Autodesk Fusion 360 part; units mm, degrees
note: some values were not read from the file. Chosen so that the rebuilt part matches the saved one: which bodies a step acts on. Set by a fixed rule: which sketch regions a step uses.
(part 3 of 3)
sketch "Sketch8" plane through (0, 0.6486, 0) normal (0, 1, 0) x (1, 0, 0)
  line L0 (0.635, 0) -> (-0.635, 0)
  line L1 (-0.635, 0) -> (-0.635, 1.947)
  line L2 (-0.635, 1.947) -> (0.635, 1.947)
  line L3 (0.635, 1.947) -> (0.635, 0)
  line L4 (0.1879, 0.6932) -> (0.1773, 0.6456)
  line L5 (-0.3149, 1.0213) -> (-0.3096, 1.0054)
  line L6 (-0.3307, 0.5821) -> (-0.3254, 0.6085)
  line L7 (-0.4948, 0.598) -> (-0.8334, 0.2593)
  line L8 (-0.1773, 0.5556) -> (-0.172, 0.598)
  line L9 (-0.3254, 0.6297) -> (-0.3307, 0.6509)
  line L10 (-0.4101, 0) -> (-0.2831, 0.1005)
  line L11 (-0.4683, 1.0425) -> (-0.4683, 1.0054)
  line L12 (-0.2831, 0.1005) -> (-0.2831, 0.2064)
  line L13 (-0.2778, 0.3069) -> (-0.1931, 0.508)
  line L14 (-0.172, 0.6456) -> (-0.1826, 0.6932)
  line L15 (-0.4207, 0.3598) -> (-0.2778, 0.3069)
  line L16 (-0.4683, 1.0054) -> (-0.4577, 0.9631)
  line L17 (-0.3149, 1.0425) -> (-0.3149, 1.0213)
  line L18 (-0.336, 0.5609) -> (-0.3307, 0.5821)
  line L19 (13.8033, 2.0479) -> (13.8033, 2.3548)
  line L20 (0.4207, 2.8522) -> (0.4207, 2.5347)
  line L21 (0.3836, 2.8152) -> (0.4207, 2.8522)
  line L22 (0.4948, 2.8628) -> (0.4789, 2.8734)
  line L23 (13.5229, 2.831) -> (13.5229, 2.8416)
  line L24 (0.9075, 2.9686) -> (1.0081, 2.7675)
  line L25 (13.6022, 2.7675) -> (13.6022, 2.4871)
  line L26 (0.8811, 2.8522) -> (0.9181, 2.8152)
  line L27 (13.5811, 2.7675) -> (13.6022, 2.7675)
  line L28 (0.5689, 2.9686) -> (0.3942, 2.9686)
  line L29 (0.5054, 2.8416) -> (0.4948, 2.8628)
  line L30 (0.8811, 2.8522) -> (0.8811, 2.5347)
  line L31 (13.6022, 2.323) -> (13.6022, 2.0479)
  line L32 (13.5281, 2.3548) -> (13.5281, 2.0479)
  line L33 (13.5281, 2.8205) -> (13.5281, 2.5135)
  line L34 (1.0081, 2.7675) -> (0.9763, 2.7675)
  line L35 (0.5847, 2.7675) -> (0.5636, 2.7675)
  line L36 (0.8387, 2.8787) -> (0.8229, 2.8734)
  line L37 (0.336, 2.7675) -> (0.3254, 2.7675)
  line L38 (13.4805, 2.8787) -> (13.4964, 2.8734)
  line L39 (13.8086, 2.8416) -> (13.8033, 2.831)
  line L40 (0.7382, 2.7675) -> (0.717, 2.7675)
  line L41 (0.4789, 2.8734) -> (0.463, 2.8787)
  line L42 (13.8086, 2.3654) -> (13.8086, 2.0479)
  line L43 (13.507, 2.8628) -> (13.5229, 2.8416)
  line L44 (13.4382, 2.8522) -> (13.4382, 2.5347)
  line L45 (0.5054, 2.8416) -> (0.5159, 2.8205)
  line L46 (0.3254, 2.7675) -> (0.3254, 2.4871)
  line L47 (0.5265, 2.7993) -> (0.5159, 2.8205)
  line L48 (13.3482, 2.7675) -> (13.3641, 2.7781)
  line L49 (0.9763, 2.0479) -> (0.9763, 2.323)
  line L50 (2.3892, 2.2013) -> (2.3892, 2.0479)
  line L51 (1.5161, 2.0479) -> (1.5161, 2.2013)
  line L52 (13.9674, 2.7781) -> (13.9832, 2.7675)
  line L53 (4.1196, 2.2013) -> (4.1196, 2.0479)
  line L54 (13.3376, 2.4871) -> (13.3376, 2.7675)
  line L55 (6.7231, 2.0479) -> (6.2944, 2.0479)
  line L56 (0.5054, 2.8416) -> (0.5054, 2.5241)
  line L57 (7.5962, 2.2013) -> (7.5962, 2.0479)
  line L58 (1.0874, 2.2013) -> (1.0874, 2.0479)
  line L59 (2.8178, 2.2013) -> (2.3892, 2.2013)
  line L60 (7.157, 1.4129) -> (7.157, 2.4395)
  line L61 (0.717, 2.7675) -> (0.5847, 2.7675)
  line L62 (1.5161, 2.2013) -> (1.0874, 2.2013)
  line L63 (8.0248, 2.2013) -> (7.5962, 2.2013)
  line L64 (13.3059, 2.4871) -> (13.3059, 2.7675)
  line L65 (10.6283, 2.2013) -> (10.1944, 2.2013)
  line L66 (0.4207, 2.3707) -> (0.4207, 2.0479)
  line L67 (0.8811, 2.3707) -> (0.8811, 2.0479)
  line L68 (2.8178, 2.0479) -> (2.8178, 2.2013)
  line L69 (0.5159, 2.0479) -> (0.5159, 2.3548)
  line L70 (0.3254, 2.323) -> (0.3254, 2.0479)
  line L71 (13.5229, 2.8416) -> (13.5229, 2.5241)
  line L72 (13.3059, 2.7675) -> (13.3376, 2.7675)
  line L73 (0.7858, 2.8205) -> (0.7858, 2.5135)
  line L74 (0.7964, 2.3654) -> (0.7964, 2.0479)
  line L75 (6.7231, 2.2013) -> (6.7231, 2.0479)
  line L76 (11.4961, 2.0479) -> (11.4961, 2.2013)
  line L77 (0.717, 1.8097) -> (0.5001, 1.5928)
  line L78 (0.7911, 1.5187) -> (0.6535, 2.0479)
  line L79 (0.717, 2.323) -> (0.717, 2.0479)
  line L80 (0.3836, 2.3495) -> (0.3836, 2.0479)
  line L81 (10.6283, 2.0479) -> (10.1944, 2.0479)
  line L82 (5.4213, 2.2013) -> (4.9927, 2.2013)
  line L83 (0.5159, 2.5135) -> (0.5159, 2.8205)
  line L84 (13.4117, 2.9686) -> (13.5864, 2.9686)
  line L85 (13.3376, 2.0479) -> (13.3376, 2.323)
  line L86 (8.0248, 2.0479) -> (7.5962, 2.0479)
  line L87 (13.4594, 2.8734) -> (13.4805, 2.8787)
  line L88 (4.1196, 2.0479) -> (3.6909, 2.0479)
  line L89 (3.6909, 2.2013) -> (3.6909, 2.0479)
  line L90 (0.5054, 2.3654) -> (0.5054, 2.0479)
  line L91 (13.3376, 2.7675) -> (13.3482, 2.7675)
  line L92 (0.9181, 2.0479) -> (0.9181, 2.3495)
  line L93 (0.7858, 2.3548) -> (0.7858, 2.0479)
  line L94 (13.7716, 2.7781) -> (13.8033, 2.8205)
  line L95 (1.0081, 2.0479) -> (1.0081, 2.323)
  line L96 (0.8229, 2.8734) -> (0.807, 2.8628)
  line L97 (13.2318, 2.2013) -> (12.7979, 2.2013)
  line L98 (12.7979, 2.2013) -> (12.7979, 2.0479)
  line L99 (13.5229, 2.3654) -> (13.5229, 2.0479)
  line L100 (13.4011, 2.0479) -> (13.4011, 2.3495)
  line L101 (13.8086, 2.8416) -> (13.8086, 2.5241)
  line L102 (8.8979, 2.2013) -> (9.3266, 2.2013)
  line L103 (13.5281, 2.8205) -> (13.5229, 2.831)
  line L104 (0.7858, 2.8205) -> (0.7964, 2.8416)
  line L105 (0.3678, 2.794) -> (0.3519, 2.7781)
  line L106 (4.1196, 2.2013) -> (3.6909, 2.2013)
  line L107 (0.8811, 2.8522) -> (0.8599, 2.8734)
  line L108 (13.3059, 2.0479) -> (13.3059, 2.323)
  line L109 (9.3266, 2.0479) -> (8.8979, 2.0479)
  line L110 (6.2944, 2.2013) -> (6.2944, 2.0479)
  line L111 (13.7504, 2.7675) -> (13.7716, 2.7781)
  line L112 (13.2318, 2.0479) -> (12.7979, 2.0479)
  line L113 (0.3836, 2.8152) -> (0.3678, 2.794)
  line L114 (13.6022, 2.7675) -> (13.7292, 2.7675)
  line L115 (0.9763, 2.4871) -> (0.9763, 2.7675)
  line L116 (0.717, 2.7675) -> (0.717, 2.4871)
  line L117 (0.3836, 2.8152) -> (0.3836, 2.5135)
  line L118 (0.7594, 2.7781) -> (0.7382, 2.7675)
  line L119 (13.4382, 2.3707) -> (13.4382, 2.0479)
  line L120 (0.9181, 2.5135) -> (0.9181, 2.8152)
  line L121 (13.8033, 2.5135) -> (13.8033, 2.8205)
  line L122 (13.4011, 2.5135) -> (13.4011, 2.8152)
  line L123 (13.8033, 2.831) -> (13.8033, 2.8205)
  line L124 (0.9657, 2.7675) -> (0.9181, 2.8152)
  line L125 (0.463, 2.8787) -> (0.4419, 2.8681)
  line L126 (13.4382, 2.8522) -> (13.4594, 2.8734)
  line L127 (11.9301, 2.0479) -> (11.4961, 2.0479)
  line L128 (13.2318, 2.2013) -> (13.2318, 2.0479)
  line L129 (0.807, 2.8628) -> (0.7964, 2.8416)
  line L130 (1.0081, 2.4871) -> (1.0081, 2.7675)
  line L131 (0.9075, 2.9686) -> (0.7329, 2.9686)
  line L132 (13.544, 2.7993) -> (13.5599, 2.7781)
  line L133 (13.7292, 2.7675) -> (13.7504, 2.7675)
  line L134 (0.5477, 2.7781) -> (0.5265, 2.7993)
  line L135 (0.3519, 2.7781) -> (0.336, 2.7675)
  line L136 (13.417, 2.8363) -> (13.4011, 2.8152)
  line L137 (0.7752, 2.7993) -> (0.7594, 2.7781)
  line L138 (13.8086, 2.8416) -> (13.8245, 2.8628)
  line L139 (0.4419, 2.8681) -> (0.4207, 2.8522)
  line L140 (0.9763, 2.7675) -> (0.9657, 2.7675)
  line L141 (13.4964, 2.8734) -> (13.507, 2.8628)
  line L142 (13.4382, 2.8522) -> (13.417, 2.8363)
  line L143 (13.5599, 2.7781) -> (13.5811, 2.7675)
  line L144 (0.7964, 2.8416) -> (0.7964, 2.5241)
  line L145 (0.5636, 2.7675) -> (0.5477, 2.7781)
  line L146 (0.7858, 2.8205) -> (0.7752, 2.7993)
  line L147 (13.5281, 2.8205) -> (13.544, 2.7993)
  line L148 (0.8599, 2.8734) -> (0.8387, 2.8787)
  line L149 (0.3201, 1.0425) -> (0.3201, 1.8415)
  line L150 (-0.4948, 1.6827) -> (-0.8334, 1.3494)
  line L151 (0.2831, 0.1005) -> (0.2831, 0.2064)
  line L152 (-0.336, 0.5609) -> (-0.4207, 0.3598)
  line L153 (0.2778, 0.3069) -> (0.1931, 0.508)
  line L154 (0.5001, 0.2064) -> (0.5001, 1.9473)
  line L155 (-0.8334, 0) -> (-0.8334, 2.0479)
  line L156 (15.1527, 2.0479) -> (15.1527, 0)
  line L157 (-0.463, 0.9684) -> (-0.3307, 0.6509)
  line L158 (-0.4948, 1.3229) -> (-0.8334, 0.9843)
  line L159 (-0.1879, 0.508) -> (-0.1773, 0.5556)
  line L160 (-0.3254, 0.6085) -> (-0.3254, 0.6297)
  line L161 (-0.4948, 0.9631) -> (-0.8334, 0.6244)
  line L162 (-0.1826, 0.6932) -> (-0.3096, 1.0054)
  line L163 (-0.172, 0.598) -> (-0.172, 0.6456)
  line L164 (0.1773, 0.598) -> (0.1826, 0.5556)
  line L165 (0.1773, 0.6456) -> (0.1773, 0.598)
  line L166 (0.2831, 0.1005) -> (-0.2831, 0.1005)
  line L167 (-0.3149, 1.2806) -> (-0.4683, 1.2806)
  line L168 (-0.4948, 0.2381) -> (-0.7329, 0)
  line L169 (0.1826, 0.5556) -> (0.1931, 0.508)
  line L170 (0.336, 0.6509) -> (0.3307, 0.6297)
  line L171 (7.157, -0.381) -> (7.157, 0.6456)
  line L172 (-0.4948, 0.2064) -> (-0.4948, 1.9473)
  line L173 (0.7911, 1.524) -> (0.5001, 1.2277)
  line L174 (0.6482, 0.5345) -> (0.7911, 1.5187)
  line L175 (0.4736, 1.8415) -> (0.4736, 1.0425)
  line L176 (0.3201, 1.0213) -> (0.3201, 1.0425)
  line L177 (13.8245, 2.8628) -> (13.8351, 2.8734)
  line L178 (0.6694, 0.6773) -> (0.5001, 0.508)
  line L179 (-0.3149, 1.0425) -> (-0.3149, 1.8415)
  line L180 (0.336, 0.5821) -> (0.3413, 0.5609)
  line L181 (0.4101, 0) -> (0.2831, 0.1005)
  line L182 (15.1527, 1.9473) -> (0.68, 1.9473)
  line L183 (0.463, 0.9684) -> (0.336, 0.6509)
  line L184 (-0.4683, 1.8415) -> (-0.4683, 1.0425)
  line L185 (0.3149, 1.0054) -> (0.3201, 1.0213)
  line L186 (15.1527, 0) -> (-0.8334, 0)
  line L187 (15.1527, 2.0479) -> (0.2143, 2.0479)
  line L188 (13.7451, 2.9686) -> (13.9197, 2.9686)
  line L189 (0.4736, 1.2806) -> (0.3201, 1.2806)
  line L190 (13.9938, 2.323) -> (13.9938, 2.0479)
  line L191 (14.0256, 2.4871) -> (14.0256, 2.7675)
  line L192 (13.9144, 2.8363) -> (13.8933, 2.8522)
  line L193 (0.2937, 2.0479) -> (0.2937, 2.323)
  line L194 (0.7329, 0) -> (0.6482, 0.5345)
  line L195 (0.2143, 2.2013) -> (0.2143, 1.8415)
  line L196 (0.1826, 0.6932) -> (0.3149, 1.0054)
  line L197 (0.3201, 1.1271) -> (-0.3149, 1.1271)
  line L198 (0.7329, 1.1007) -> (0.5001, 0.8678)
  line L199 (7.157, 0.8996) -> (7.157, 1.1589)
  line L200 (0.7276, 0.0106) -> (0.717, 0)
  line L201 (0.5001, 0.2064) -> (-0.4948, 0.2064)
  line L202 (0.4207, 0.3598) -> (0.2778, 0.3069)
  line L203 (0.68, 0.3228) -> (0.3784, 0.0265)
  line L204 (-0.6482, 1.8944) -> (-0.8334, 1.7092)
  line L205 (0.3307, 0.6085) -> (0.336, 0.5821)
  line L206 (0.4736, 1.0054) -> (0.4736, 1.0425)
  line L207 (0.463, 0.9631) -> (0.4736, 1.0054)
  line L208 (14.5336, 2.0479) -> (14.5336, 2.2013)
  line L209 (13.8933, 2.8522) -> (13.8933, 2.5347)
  line L210 (14.5336, 2.2013) -> (14.0996, 2.2013)
  line L211 (13.8562, 2.8787) -> (13.8721, 2.8681)
  line L212 (13.9938, 2.7675) -> (13.9938, 2.4871)
  line L213 (-0.2143, 2.0479) -> (0.2143, 2.0479)
  line L214 (0.3307, 0.6297) -> (0.3307, 0.6085)
  line L215 (0.336, 0.5609) -> (0.4207, 0.3598)
  line L216 (0.3254, 2.7675) -> (0.2937, 2.7675)
  line L217 (13.9197, 2.9686) -> (14.0256, 2.7675)
  line L218 (9.3266, 2.2013) -> (9.3266, 2.0479)
  line L219 (14.5336, 2.0479) -> (14.0996, 2.0479)
  line L220 (14.0996, 2.2013) -> (14.0996, 2.0479)
  line L221 (13.9303, 2.8152) -> (13.9144, 2.8363)
  line L222 (14.0256, 2.0479) -> (14.0256, 2.323)
  line L223 (8.8979, 2.2013) -> (8.8979, 2.0479)
  line L224 (0.2937, 2.4871) -> (0.2937, 2.7675)
  line L225 (0.3942, 2.9686) -> (0.2937, 2.7675)
  line L226 (-0.2143, 1.8415) -> (-0.4683, 1.8415)
  line L227 (0.68, 1.9473) -> (0.2143, 1.9473)
  line L228 (5.4213, 2.0479) -> (5.4213, 2.2013)
  line L229 (4.9927, 2.2013) -> (4.9927, 2.0479)
  line L230 (0.2143, 1.8415) -> (0.4736, 1.8415)
  line L231 (-0.2143, 1.8415) -> (-0.2143, 2.2013)
  line L232 (13.8933, 2.3707) -> (13.8933, 2.0479)
  line L233 (-0.2143, 1.9473) -> (-0.8334, 1.9473)
  line L234 (-0.2143, 2.2013) -> (0.2143, 2.2013)
  line L235 (13.8351, 2.8734) -> (13.8562, 2.8787)
  line L236 (-0.2143, 2.0479) -> (-0.8334, 2.0479)
  line L237 (13.9303, 2.3495) -> (13.9303, 2.0479)
  line L238 (11.9301, 2.2013) -> (11.4961, 2.2013)
  line L239 (11.9301, 2.0479) -> (11.9301, 2.2013)
  line L240 (13.9938, 2.7675) -> (14.0256, 2.7675)
  line L241 (13.3641, 2.7781) -> (13.4011, 2.8152)
  line L242 (13.4117, 2.9686) -> (13.3059, 2.7675)
  line L243 (10.6283, 2.0479) -> (10.6283, 2.2013)
  line L244 (13.9832, 2.7675) -> (13.9938, 2.7675)
  line L245 (13.9303, 2.8152) -> (13.9303, 2.5135)
  line L246 (13.8721, 2.8681) -> (13.8933, 2.8522)
  line L247 (2.8178, 2.0479) -> (2.3892, 2.0479)
  line L248 (8.0248, 2.0479) -> (8.0248, 2.2013)
  line L249 (13.9515, 2.794) -> (13.9674, 2.7781)
  line L250 (1.0874, 2.0479) -> (1.5161, 2.0479)
  line L251 (5.4213, 2.0479) -> (4.9927, 2.0479)
  line L252 (6.2944, 2.2013) -> (6.7231, 2.2013)
  line L253 (13.9303, 2.8152) -> (13.9515, 2.794)
  line L254 (10.1944, 2.0479) -> (10.1944, 2.2013)
  line L255 (0, 2.2013) -> (0, 0)
  line L256 (0.463, 0.9684) -> (0.4736, 1.0054)
  line L257 (0.1879, 0.6932) -> (0.1951, 0.7229)
  line L258 (0.3413, 0.5609) -> (0.345, 0.5395)
  constraint midpoint L234 L255.start
  constraint coincident L186 L255.end
  constraint perpendicular L186 L255
  constraint coincident L183.start L256.start
  constraint coincident L206.start L207.end
  constraint coincident L4.start L257.start
  constraint coincident L196 L257.end
  constraint coincident L180.end L258.start
  constraint coincident L215 L258.end
sketch "Sketch9" plane through (0, 0, 0) normal (0, 0, 1) x (1, 0, 0)
  line L0 (0, 0.392) -> (0, 0.9053)
  line L1 (0.2831, 0.6486) -> (-0.2831, 0.6486)
  line L2 (-0.2831, 0.392) -> (0.2831, 0.392)
  line L3 (0.2831, 0.392) -> (0.2831, 0.9053)
  line L4 (0.2831, 0.9053) -> (-0.2831, 0.9053)
  line L5 (-0.2831, 0.9053) -> (-0.2831, 0.392)
  line L6 (0, 0.2809) -> (0, 1.1222)
  line L7 (0.5001, 0.6486) -> (-0.4948, 0.6486)
  line L8 (-0.4948, 0.2809) -> (0.5001, 0.2809)
  line L9 (0.5001, 0.2809) -> (0.5001, 1.1222)
  line L10 (0.5001, 1.1222) -> (-0.4948, 1.1222)
  line L11 (-0.4948, 1.1222) -> (-0.4948, 0.2809)
  constraint horizontal L2
  constraint vertical L3
  constraint horizontal L4
  constraint vertical L5
  constraint coincident L1.end L5
  constraint coincident L0.end L4
  constraint coincident L1.start L3
  constraint coincident L0.start L2
  constraint horizontal L8
  constraint vertical L9
  constraint horizontal L10
  constraint vertical L11
  constraint coincident L7.end L11
  constraint coincident L6.end L10
  constraint coincident L7.start L9
  constraint coincident L6.start L8
extrude "Extrude3" cut sketch "Sketch9" against normal up to surface (0.2064 mm away) contours L0 L1 L2 L5 L6 L7 | L0 L1 L2 L3 L6 L7 | L0 L1 L4 L5 L6 L7 | L0 L1 L3 L4 L6 L7 bodies 1
extrude "Extrude4" cut sketch "Sketch9" against normal up to surface (1.741 mm away) from surface at -0.2064 bodies 1
chamfer "Chamfer2" distance 0.153 distance2 0.101 4 edges at (0, 0.9053, 0) (0.2831, 0.6486, 0) (0, 0.392, 0) (-0.2831, 0.6486, 0) measured on face at (0.0944, 1.3251, 0) measured on face at (0.0944, 1.3251, 0) measured on face at (0.0944, 1.3251, 0) measured on face at (0.0944, 1.3251, 0) on bodies 1
sketch "Sketch10" plane through (0, 0, 0) normal (1, 0, 0) x (0, 1, 0)
  line L0 (2.5616, -2.0479) -> (2.5616, -2.2013)
  line L1 (1.2016, -2.2013) -> (2.5616, -2.2013)
  line L2 (2.5616, -2.2013) -> (1.2016, -2.2013)
  line L3 (2.5616, -2.0479) -> (1.2016, -2.0479)
  line L4 (2.5616, -2.0479) -> (1.2016, -2.0479)
  arc A0 (1.1222, -1.9473) -> (1.2228, -2.0479) centre (1.2228, -1.9473) ccw
  line L5 (1.1222, -1.9685) -> (1.1222, -1.1271)
  arc A1 (0.9688, -1.947) -> (1.2231, -2.2013) centre (1.2231, -1.947) ccw
  line L6 (0.9688, -1.8415) -> (0.9688, -1.9685)
  line L7 (0, -1.947) -> (1.535, -1.947)
  point P0 (2.5616, -2.0479)
  point P1 (2.5616, -2.2013)
  point P2 (1.2016, -2.2013)
  point P3 (1.2016, -2.0479)
  point P4 (1.1222, -1.9473)
  point P5 (0.9688, -1.8415)
  constraint coincident P0 L0.start
  constraint coincident P1 L0.end
  constraint coincident P2 L1.start
  constraint coincident P3 L3.end
  constraint tangent L3 A0
  constraint coincident P4 A0.start
  constraint coincident L3 A0.end
  constraint tangent A0 L5
  constraint coincident A1.start L6
  constraint coincident A1.start L7
  constraint coincident L1 A1.end
  constraint tangent L1 A1
  constraint tangent A1 L6
extrude "Extrude6" add sketch "Sketch10" along normal mid plane 0.42 separate body makes body 2
extrude "Extrude7" add sketch "Sketch8" along normal up to surface (0.4736 mm away) and the other way up to surface (0.3678 mm away) separate body contours L4 L149 L153 L164 L165 L169 L170 L175 L176 L180 L183 L185 L189 L196 L202 L205 L206 L207 L214 L215 L256 L257 L258 | L149 L175 L189 L230 makes body 3
extrude "Extrude8" cut sketch "Sketch7" along normal blind 1.1 contours L5 L14 L16 L18 L23 L24 L32 L34 L42 L48 L53 L121 L124 L129 L146 L148 L151 L170 L174 L182 L199 L261 L274 L284 L293 L294 | L2 L14 L51 L54 L79 L84 L91 L93 L97 L132 L133 L138 L141 L152 L161 L242 L291 L292 bodies 3
mirror "Mirror1" about plane through (0, 0, 0) normal (1, 0, 0) of bodies 3 makes body 4
pattern_linear "R-Pattern1" count 11 spacing 1.27 along (1, 0, 0) of bodies 3 1 4 2 makes body 5 at (0.635, 0.5117, -0.649) makes body 6 at (2.7517, 0, -0.649) makes body 7 at (4.0217, 0, -0.649) makes body 8 at (5.2917, 0, -0.649) makes body 9 at (6.5617, 0, -0.649) makes body 10 at (7.8317, 0, -0.649) makes body 11 at (9.1017, 0, -0.649) makes body 12 at (10.3717, 0, -0.649) makes body 13 at (11.6417, 0, -0.649) makes body 14 at (13.335, 1.0233, -0.649) makes body 15 at (1.34, 2.1153, -2.0479) makes body 16 at (2.61, 2.1153, -2.0479) makes body 17 at (3.88, 2.1153, -2.0479) makes body 18 at (5.15, 2.1153, -2.0479) makes body 19 at (6.42, 2.1153, -2.0479) makes body 20 at (7.69, 2.1153, -2.0479) makes body 21 at (8.96, 2.1153, -2.0479) makes body 22 at (10.23, 2.1153, -2.0479) makes body 23 at (11.5, 2.1153, -2.0479) makes body 24 at (12.77, 2.1153, -2.0479) makes body 25 at (1.5901, 0.9132, -1.4676) makes body 26 at (2.8601, 0.9132, -1.4676) makes body 27 at (4.1301, 0.9132, -1.4676) makes body 28 at (5.4001, 0.9132, -1.4676) makes body 29 at (6.6701, 0.9132, -1.4676) makes body 30 at (7.9401, 0.9132, -1.4676) makes body 31 at (9.2101, 0.9132, -1.4676) makes body 32 at (10.4801, 0.9132, -1.4676) makes body 33 at (11.7501, 0.9132, -1.4676) makes body 34 at (13.0201, 0.9132, -1.4676) makes body 35 at (0.9499, 0.9132, -1.4676) makes body 36 at (2.2199, 0.9132, -1.4676) makes body 37 at (3.4899, 0.9132, -1.4676) makes body 38 at (4.7599, 0.9132, -1.4676) makes body 39 at (6.0299, 0.9132, -1.4676) makes body 40 at (7.2999, 0.9132, -1.4676) makes body 41 at (8.5699, 0.9132, -1.4676) makes body 42 at (9.8399, 0.9132, -1.4676) makes body 43 at (11.1099, 0.9132, -1.4676) makes body 44 at (12.3799, 0.9132, -1.4676)
mirror "Mirror2" about plane through (0, 0, 0) normal (0, 1, 0) of bodies 1 3 2 4 6 5 7 8 9 11 12 10 16 19 14 13 15 17 18 20 21 22 23 27 25 24 26 31 28 29 30 33 34 32 35 39 41 37 44 36 38 40 42 43 makes body 45 at (-0.635, -0.5117, -0.649) makes body 46 at (0.07, -2.1153, -2.0479) makes body 47 at (0.3201, -0.9132, -1.4676) makes body 48 at (-0.3201, -0.9132, -1.4676) makes body 49 at (1.4817, 0, -0.649) makes body 50 at (2.7517, 0, -0.649) makes body 51 at (4.0217, 0, -0.649) makes body 52 at (5.2917, 0, -0.649) makes body 53 at (6.5617, 0, -0.649) makes body 54 at (7.8317, 0, -0.649) makes body 55 at (9.1017, 0, -0.649) makes body 56 at (10.3717, 0, -0.649) makes body 57 at (11.6417, 0, -0.649) makes body 58 at (13.335, -1.0233, -0.649) makes body 59 at (1.34, -2.1153, -2.0479) makes body 60 at (2.61, -2.1153, -2.0479) makes body 61 at (3.88, -2.1153, -2.0479) makes body 62 at (5.15, -2.1153, -2.0479) makes body 63 at (6.42, -2.1153, -2.0479) makes body 64 at (7.69, -2.1153, -2.0479) makes body 65 at (8.96, -2.1153, -2.0479) makes body 66 at (10.23, -2.1153, -2.0479) makes body 67 at (11.5, -2.1153, -2.0479) makes body 68 at (12.77, -2.1153, -2.0479) makes body 69 at (1.5901, -0.9132, -1.4676) makes body 70 at (2.8601, -0.9132, -1.4676) makes body 71 at (4.1301, -0.9132, -1.4676) makes body 72 at (5.4001, -0.9132, -1.4676) makes body 73 at (6.6701, -0.9132, -1.4676) makes body 74 at (7.9401, -0.9132, -1.4676) makes body 75 at (9.2101, -0.9132, -1.4676) makes body 76 at (10.4801, -0.9132, -1.4676) makes body 77 at (11.7501, -0.9132, -1.4676) makes body 78 at (13.0201, -0.9132, -1.4676) makes body 79 at (0.9499, -0.9132, -1.4676) makes body 80 at (2.2199, -0.9132, -1.4676) makes body 81 at (3.4899, -0.9132, -1.4676) makes body 82 at (4.7599, -0.9132, -1.4676) makes body 83 at (6.0299, -0.9132, -1.4676) makes body 84 at (7.2999, -0.9132, -1.4676) makes body 85 at (8.5699, -0.9132, -1.4676) makes body 86 at (9.8399, -0.9132, -1.4676) makes body 87 at (11.1099, -0.9132, -1.4676) makes body 88 at (12.3799, -0.9132, -1.4676)
combine "Combine1" operation add target body 1 tool bodies 5 45 49 50 6 7 51 52 53 9 8 10 12 11 13 14 57 58 56 55 54
move_face "OffsetFaces1" offset 0.12 2 faces at (13.335, 0.5117, -0.649) (-0.635, -0.5117, -0.649) on bodies 1
